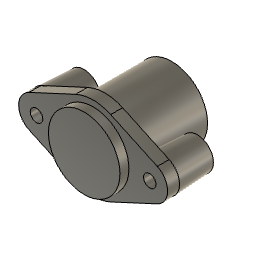
BLS_Griff_ausV1 (Autodesk Fusion 360 archive; units mm, degrees)
design "230322_Mini-DIN_Buchse"
Autodesk Fusion 360 part; units mm, degrees
sketch "Skizze1" plane through (0, 0, 0) normal (0, 1, 0) x (1, 0, 0)
  circle A0 centre (0, 0) radius 6
  circle A1 centre (0, 0) radius 7
  line L0 (0, -25) -> (0, 25) construction
  line L1 (-50, 0) -> (45, 0) construction
  circle A2 centre (-9.5, 0) radius 1.05
  circle A3 centre (-9.5, 0) radius 3
  line L2 (-2.9474, -6.3493) -> (-10.7632, -2.7211)
  line L3 (-2.9474, 6.3493) -> (-10.7632, 2.7211)
  circle A4 centre (9.5, 0) radius 3
  circle A5 centre (9.5, 0) radius 1.05
  line L4 (2.9474, -6.3493) -> (10.7632, -2.7211)
  line L5 (2.9474, 6.3493) -> (10.7632, 2.7211)
  circle A6 centre (0, 0) radius 5.5
  dimension "d1" = 12
  dimension "d2" = 14
  dimension "d3" = 2.1
  dimension "d4" = 9.5
  dimension "d5" = 6
  dimension "d6" = 11
  constraint coincident A0.centre A1.centre
  constraint vertical L0
  constraint horizontal L1
  constraint coincident L1 A2.centre
  constraint concentric A2 A3
  constraint coincident A1 L2.start
  constraint tangent A1 L2
  constraint tangent A3 L2
  constraint coincident A3 L2.end
  constraint symmetric L1 L2.start L3.start
  constraint symmetric L1 L2.end L3.end
  constraint symmetric L0 A2 A5
  constraint symmetric L0 A3 A4
  constraint symmetric L0 L2.start L4.start
  constraint symmetric L0 L2.end L4.end
  constraint symmetric L0 L3.start L5.start
  constraint symmetric L0 L3.end L5.end
  constraint concentric A0 A6
  measures "d1" diameter of A0
  measures "d2" diameter of A1
  measures "d3" diameter of A2
  measures "d4" distance of L0 A2.centre
  measures "d5" diameter of A3
  measures "d6" diameter of A6
extrude "Extrusion1" add sketch "Skizze1" along normal blind 6 draft -3 contours A1 A4 | A1 A4 | A1 A3 | A1 A3 makes body 1 at (8.4231, 1, 2.7438) makes body 2 at (-10.5769, 1, 2.7438)
extrude "Extrusion2" add sketch "Skizze1" along normal blind 11.2 separate body contours A0 | A6 makes body 3
extrude "Extrusion3" add sketch "Skizze1" against normal blind 2 contours A0 | A1 A3 A4 | A1 A4 L5 | A1 A3 L3 | A1 A4 | A1 A4 | A1 A3 | A1 A3 | A1 A4 L4 | A1 A3 L2 | A6 bodies 1 2 3
extrude "Extrusion4" add sketch "Skizze1" against normal blind 3.5 contours A0 | A6 bodies 1
